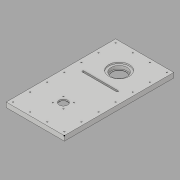
# Autodesk Inventor part: b_base_cover_1
Saved by Autodesk Inventor 2019 (Build 230136000, 136)
## iProperties
Created: 2021-11-06
Part Number: b_base_cover_1
Material: Generic
Document SubType Name: Modeling
Designer: Mohamed
Density: 1 g/cm^3
Appearance: Default
Author: Mohamed
Autodesk Inventor part; units mm, degrees
ref_plane "YZ Plane" through (0, 0, 0) normal (1, 0, 0) x (0, 1, 0)
ref_plane "XZ Plane" through (0, 0, 0) normal (0, 1, 0) x (-1, 0, 0)
ref_plane "XY Plane" through (0, 0, 0) normal (0, 0, 1) x (1, 0, 0)
sketch "Sketch1" plane through (0, 0, 0) normal (0, 1, 0) x (-1, 0, 0)
  line L0 (0, 0) -> (170, 0)
  line L1 (170, 0) -> (170, -320)
  line L2 (170, -320) -> (0, -320)
  line L3 (0, -320) -> (0, 0)
  dimension "d0" = 170
  dimension "d1" = 320
  constraints: 8 end point, 2 parallel, 1 horizontal, 1 perpendicular
  measures "d0" distance of L1.end L2.end
  measures "d1" distance of L0.end L1.end
extrude "Extrusion1" add sketch "Sketch1" along normal blind 14
sketch "Sketch2" plane through (0, 14, 0) normal (0, 1, 0) x (1, 0, 0)
  line L0 (0, 320) -> (-170, 320) projected
  circle A0 centre (-85, 245) radius 30
  point P0 (0, 0)
  dimension "d5" = 60
  constraints: 1 centre point
  measures "d5" diameter of A0
extrude "Extrusion2" cut sketch "Sketch2" against normal blind 4
sketch "Sketch3" plane through (-85, 10, -245) normal (0, 1, 0) x (1, 0, 0)
  circle A0 centre (0, 0) radius 23.5
  point P0 (85, -245)
  dimension "d8" = 47
  constraints: 1 centre point
  measures "d8" diameter of A0
extrude "Extrusion3" cut sketch "Sketch3" against normal blind 9
sketch "Sketch4" plane through (-85, 1, -245) normal (0, 1, 0) x (1, 0, 0)
  circle A0 centre (0, 0) radius 20
  point P0 (85, -245)
  dimension "d11" = 40
  constraints: 1 centre point
  measures "d11" diameter of A0
extrude "Extrusion4" cut sketch "Sketch4" against normal blind 1
sketch "Sketch5" plane through (0, 14, 0) normal (0, 1, 0) x (1, 0, 0)
  circle A0 centre (-85, 245) radius 30 projected
  circle A1 centre (-85, 82.3) radius 12.5
  circle A2 centre (-100.5, 66.8) radius 1.6
  circle A3 centre (-100.5, 97.8) radius 1.6
  circle A4 centre (-69.5, 97.8) radius 1.6
  circle A5 centre (-69.5, 66.8) radius 1.6
  point P0 (0, 0)
  dimension "d15" = 25
  dimension "d22" = 3.2
  dimension "d23" = 3.2
  dimension "d24" = 3.2
  dimension "d25" = 3.2
  constraints: 5 centre point
  measures "d15" diameter of A1
  measures "d22" diameter of A2
  measures "d23" diameter of A3
  measures "d24" diameter of A4
  measures "d25" diameter of A5
extrude "Extrusion5" cut sketch "Sketch5" against normal blind 14 contours A1 | A2 | A3 | A4 | A5
sketch "Sketch6" plane through (0, 0, 0) normal (0, -1, 0) x (1, 0, 0)
  circle A0 centre (-85, -82.3) radius 12.5 projected
  line L0 (-106.5, -103.8) -> (-63.5, -103.8)
  line L1 (-63.5, -103.8) -> (-63.5, -60.8)
  line L2 (-63.5, -60.8) -> (-106.5, -60.8)
  line L3 (-106.5, -60.8) -> (-106.5, -103.8)
  point P0 (0, 0)
  dimension "d30" = 43
  dimension "d31" = 43
  constraints: 8 end point, 2 parallel, 1 horizontal, 1 perpendicular
  measures "d30" distance of L2.end L1.end
  measures "d31" distance of L1.end L0.end
extrude "Extrusion6" cut sketch "Sketch6" against normal blind 10
sketch "Sketch7" plane through (0, 0, 0) normal (0, -1, 0) x (1, 0, 0)
  circle A0 centre (-85, -82.3) radius 12.5 projected
  line L0 (-85, -187.3) -> (-35, -187.3)
  line L1 (-35, -192.3) -> (-135, -192.3)
  line L2 (-135, -187.3) -> (-85, -187.3)
  arc A1 (-135, -187.3) -> (-135, -192.3) centre (-135, -189.8) ccw
  arc A2 (-35, -192.3) -> (-35, -187.3) centre (-35, -189.8) ccw
  point P0 (0, 0)
  dimension "d34" = 105
  dimension "d36" = 5
  dimension "d37" = 100
  dimension "d38" = 5
  dimension "d39" = 5
  dimension "d40" = 5
  constraints: 6 end point, 4 point on circle, 2 centre point, 1 horizontal, 1 point on line
  measures "d34" distance of A0.centre L0.start
  measures "d36" distance of L0.end L1.start
  measures "d37" distance of L1.start L1.end
  measures "d38" distance of L1.end L2.start
  measures "d39" diameter of A1
  measures "d40" diameter of A2
extrude "Extrusion7" cut sketch "Sketch7" against normal blind 14 contours L0 A2 L1 A1 L2
sketch "Sketch8" plane through (0, 14, 0) normal (0, 1, 0) x (1, 0, 0)
  point P0 (0, 0)
sketch "Sketch9" plane through (0, 14, 0) normal (0, 1, 0) x (1, 0, 0)
  line L0 (0, 320) -> (-170, 320) projected
  line L1 (0, 320) -> (0, 310)
  line L2 (0, 0) -> (0, 320) projected
  circle A0 centre (-10, 310) radius 1.6
  line L3 (-170, 310) -> (-160, 310) construction
  circle A1 centre (-160, 310) radius 1.6
  dimension "d43" = 10
  dimension "d45" = 3.2
  dimension "d48" = 3.2
  constraints: 4 end point, 2 centre point, 1 coincident, 1 horizontal, 1 point on line
  measures "d43" distance of L0.start L1.end
  measures "d45" diameter of A0
  measures "d48" diameter of A1
extrude "Extrusion8" cut sketch "Sketch9" against normal blind 14
pattern_linear "Rectangular Pattern1" count 7 spacing 50 along (0, 0, 1) of "Extrusion8"
sketch "Sketch10" plane through (0, 14, 0) normal (0, 1, 0) x (1, 0, 0)
  circle A0 centre (-160, 310) radius 1.6 projected
  circle A1 centre (-110, 310) radius 1.6
  circle A2 centre (-160, 10) radius 1.6 projected
  circle A3 centre (-110, 10) radius 1.6
  point P0 (0, 0)
  dimension "d56" = 3.2
  dimension "d58" = 3.2
  constraints: 2 centre point
  measures "d56" diameter of A1
  measures "d58" diameter of A3
extrude "Extrusion9" cut sketch "Sketch10" against normal blind 14 contours A1 | A3
pattern_linear "Rectangular Pattern2" count 2 spacing 50 along (1, 0, 0) of "Extrusion9"
body "Solid1"
